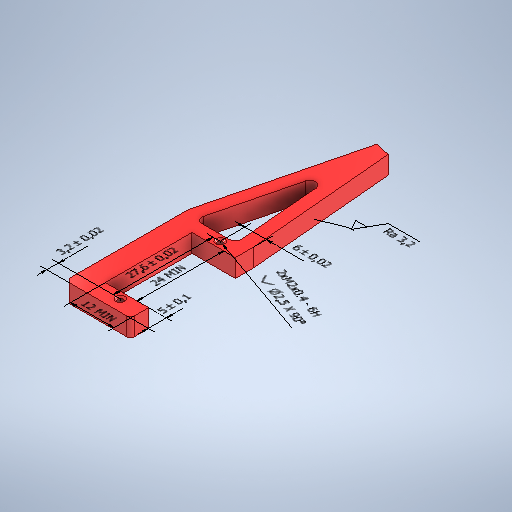
# Autodesk Inventor part: CAM3D
Saved by Autodesk Inventor 2025 (Build 290162000, 162)
## iProperties
Created: 2023-06-22
Part Number: CAM3D
Material: EN AW-6060 T6
Document SubType Name: Modeling
Designer: Roman
Density: 2.7 g/cm^3
Appearance: Light Red
Mass: 15.4015 g
Surface Area: 41.4189 cm^2
Volume: 5.70428 cm^3
Description: Přední noha
Polotovar: KR...
Author: Roman
## iProperties of the stored document CAM3D_3D tisk.ipt
Created: 2024-11-28
Part Number: CAM3D_3D tisk
Material: Všeobecné
Document SubType Name: Modeling
Designer: s21suk
Density: 1 g/cm^3
Appearance: Výchozí
Author: s21suk
## iProperties of the stored document MemberDocs/xIbcejt23Mcnw1njhJ3dlasc4Ob
Created: 2023-06-22
Part Number: CAM3D
Material: EN AW-6060 T6
Document SubType Name: Modeling
Designer: Roman
Density: 2.7 g/cm^3
Appearance: Light Red
Mass: 15.4015 g
Surface Area: 41.4189 cm^2
Volume: 5.70428 cm^3
Description: Přední noha
Polotovar: KR...
Author: Roman
Autodesk Inventor part; units mm, degrees
ref_plane "YZ Plane" through (0, 0, 0) normal (1, 0, 0) x (0, 1, 0)
ref_plane "XZ Plane" through (0, 0, 0) normal (0, 1, 0) x (-1, 0, 0)
ref_plane "XY Plane" through (0, 0, 0) normal (0, 0, 1) x (1, 0, 0)
sketch "Sketch1" plane through (0, 0, 0) normal (0, 1, 0) x (-1, 0, 0)
  line L0 (0, 0) -> (18, 0)
  line L1 (0, 0) -> (0, -5)
  line L2 (0, -5) -> (3.5719, -45.8274)
  line L3 (18, 0) -> (18, -5)
  line L4 (18, -5) -> (7.5719, -46.8247)
  line L5 (3.5719, -45.8274) -> (7.5719, -46.8247)
  dimension "d0" = 18
  dimension "d1" = 5
  dimension "d3" = 175
  dimension "d6" = 76
  dimension "d7" = 4
  constraints: 12 end point, 2 vertical, 1 horizontal, 1 parallel, 1 perpendicular
  measures "d0" distance of L0.start L0.end
  measures "d1" distance of L0.start L1.end
  measures "d3" angle of L2 L1
  measures "d6" angle of L0 L4
  measures "d7" horizontal distance of L2.end L4.end
extrude "Extrusion1" add sketch "Sketch1" along normal blind 5
shell "Shell1" thickness 3.5 removed faces 2 at (-7.1906, 5, -18.6091) at (-7.1906, 0, -18.6091)
fillet "Fillet1" radius 1.5875 5 edges at (-3.5, 2.5, -4.8472) (-6.3393, 2.5, -37.3009) (-3.5, 2.5, -3.5) (-14.5, 2.5, -3.5) (-14.5, 2.5, -4.5703)
sketch "Sketch2" plane through (0, 0, 0) normal (0, -1, 0) x (1, 0, 0)
  line L0 (0, 0) -> (-12, 0)
  line L1 (-12, 0) -> (-12, 24)
  line L2 (-12, 24) -> (0, 24)
  line L3 (0, 24) -> (0, 0)
  line L4 (0, 24) -> (-12, 24)
  line L5 (-12, 24) -> (-12, 29)
  line L6 (-12, 29) -> (0, 29)
  line L7 (0, 29) -> (0, 24)
  line L8 (-12, 0) -> (-18, 0)
  line L9 (-18, 0) -> (-18, 24)
  line L10 (-18, 24) -> (-12, 24)
  line L11 (-12, 24) -> (-12, 0)
  line L12 (-18, 24) -> (-13.7574, 24) construction
  line L13 (-12, 29) -> (-16.8, 29)
  line L14 (-16.8, 29) -> (-18, 27.8)
  line L15 (-18, 27.8) -> (-18, 24)
  dimension "d14" = 24
  dimension "d15" = 5
  dimension "d16" = 12
  dimension "d18" = 6
  dimension "d57" = 1.2
  dimension "d58" = 135
  constraints: 32 end point, 6 parallel, 5 horizontal, 4 perpendicular, 2 collinear
  measures "d14" distance of L0.end L1.end
  measures "d15" distance of L4.end L5.end
  measures "d16" distance between parallel lines of L7 L5
  measures "d18" distance between parallel lines of L9 L1
  measures "d57" horizontal distance of L14.end L13.end
  measures "d58" angle of L13 L14
extrude "Extrusion2" add sketch "Sketch2" against normal blind 5 contours L8 L9 L10 L1 | L2 L5 L6 L7 | L10 L15 L14 L13 L5
fillet "Fillet3" radius 1 1 edges at (0, 2.5, 29)
sketch "Sketch4" plane through (0, 5, 0) normal (0, 1, 0) x (1, 0, 0)
  line L0 (-12, -24) -> (-12, 0) projected
  line L1 (-12, -12) -> (-18, -12)
  line L2 (-18, 5) -> (-18, -29) projected
  line L3 (0, -24) -> (-12, -24) projected
  line L4 (-12, 0) -> (0, 0) projected
  circle A0 centre (-6, -25.8) radius 0.8
  circle A1 centre (-6, 1.8) radius 0.8
  line L5 (0, -28) -> (0, -24) projected
  point P0 (-18, 1.9304)
  point P1 (-18, -27.8)
  point P2 (-16.8, -29)
  dimension "d31" = 1.6
  dimension "d32" = 27.6
  dimension "d43" = 6
  dimension "d46" = 13.8
  constraints: 2 centre point, 2 end point, 1 horizontal, 1 midpoint, 1 symmetric about line, 3 other
  measures "d31" diameter of A0
  measures "d32" distance of A1.centre A0.centre
  measures "d43" horizontal distance of L0.start A0.centre
  measures "d46" vertical distance of A0.centre L1.end
hole "Hole1" at (-6, 5, 25.8) at (-6, 5, -1.8) direction (0, -1, 0) diameter 1.567 depth 10 countersink diameter 2.5 countersink angle 90 thread size "M2x0.4" class "6H" standard "ISO Metric profile"
sketch "Sketch17" plane through (0, 5, 0) normal (0, 1, 0) x (1, 0, 0)
  line L0 (-15.0964, 25.5) -> (0.714, 25.5)
  line L1 (-12, 0) -> (0, 0) projected
  line L2 (-5.1146, 3.5) -> (-12.7349, 3.5) projected
  line L3 (0.714, 25.5) -> (-0.9097, 44.0597)
  line L4 (-15.0964, 25.5) -> (-10.3033, 44.7241)
  line L5 (0, 5) -> (-3.5719, 45.8274) projected
  line L6 (-7.5719, 46.8247) -> (-18, 5) projected
  line L7 (-4.6811, 48.4754) -> (-4.2422, 48.3659)
  line L8 (-3.5719, 45.8274) -> (-7.5719, 46.8247) projected
  arc A0 (-0.9097, 44.0597) -> (-4.6811, 48.4754) centre (-5.8907, 43.6239) ccw
  arc A1 (-4.2422, 48.3659) -> (-10.3033, 44.7241) centre (-5.4518, 43.5145) ccw
  point P0 (-8.9248, 3.5)
  point P1 (-4.4629, 48.4157)
  dimension "d152" = 22
  dimension "d153" = 2.498
  dimension "d154" = 2.142
  dimension "d155" = 2.301
  dimension "d156" = 5
  constraints: 8 end point, 4 point on circle, 4 tangent, 3 parallel, 2 centre point, 1 equal radius, 1 horizontal, 1 midpoint
  measures "d152" distance from line of L0 point (-8.925, 3.5)
  measures "d153" distance between parallel lines of L5 L3
  measures "d154" distance between parallel lines of L4 L6
  measures "d155" distance between parallel lines of L8 L7
  measures "d156" radius of A0
extrude "Extrusion13" [suppressed]
sketch "Sketch18" plane through (-15.4653, 7.5, -25.5) normal (0, 0, 1) x (1, 0, 0)
  line L0 (16.1813, -10) -> (16.1813, 0) construction
  line L1 (4.8628, 0) -> (0, 0) construction
  line L2 (16.1813, -10) -> (0, 0) construction
  line L3 (0, -10) -> (0, 0) construction
  line L4 (16.1813, 0) -> (0, -10) construction
  line L5 (23.0907, 2.5) -> (-6.9093, 2.5)
  line L6 (-6.9093, 2.5) -> (-6.9093, -12.5)
  line L7 (-6.9093, -12.5) -> (23.0907, -12.5)
  line L8 (23.0907, -12.5) -> (23.0907, 2.5)
  line L9 (23.0907, 2.5) -> (-6.9093, -12.5) construction
  line L10 (-6.9093, 2.5) -> (23.0907, -12.5) construction
  point P0 (15.4653, -7.5)
  point P1 (8.0907, -5)
  dimension "d161" = 25
  dimension "d162" = 15
  constraints: 16 end point, 3 midpoint, 2 parallel, 1 horizontal, 1 perpendicular
  measures "d162" distance of L6.end L5.end
extrude "Extrusion14" [suppressed]
combine "Combine8" [suppressed]
extrude "Extrusion15" [suppressed]
combine "Combine9" [suppressed]
combine "Combine10" [suppressed]
sketch "Sketch20" plane through (-15.4653, 7.5, -21.5) normal (0, 0, 1) x (1, 0, 0)
  line L0 (10.1584, -7.5) -> (13.6718, -7.5) projected
  line L1 (6.1837, -2.5) -> (2.5765, -2.5) projected
  line L2 (11.871, -7.5) -> (3.871, -7.5)
  line L3 (3.871, -7.5) -> (3.871, -2.5)
  line L4 (3.871, -2.5) -> (11.871, -2.5)
  line L5 (11.871, -2.5) -> (11.871, -7.5)
  circle A0 centre (19.0907, -8.5) radius 1
  line L6 (23.0907, -12.5) -> (-6.9093, -12.5) construction
  circle A1 centre (-2.9093, -1.5) radius 1
  line L7 (23.0907, -12.5) -> (23.0907, 2.5) construction
  line L8 (23.0907, 2.5) -> (-6.9093, 2.5) construction
  line L9 (11.871, -7.5) -> (3.871, -7.5)
  line L10 (3.871, -7.5) -> (3.871, -10)
  line L11 (3.871, -10) -> (11.871, -10)
  line L12 (11.871, -10) -> (11.871, -7.5)
  line L13 (11.871, -2.5) -> (3.871, -2.5)
  line L14 (3.871, -2.5) -> (3.871, 0)
  line L15 (3.871, 0) -> (11.871, 0)
  line L16 (11.871, 0) -> (11.871, -2.5)
  line L17 (-6.9093, 2.5) -> (-6.9093, -12.5) projected
  point P0 (15.4653, -7.5)
  point P1 (23.0907, -5)
  point P2 (23.0907, -5)
  dimension "d167" = 9.224
  dimension "d168" = 3.5943
  dimension "d171" = 2
  dimension "d173" = 7.5
  dimension "d175" = 4.22
  dimension "d181" = 2.5
  dimension "d185" = 8
  dimension "d186" = 2.5
  dimension "d202" = 15
  dimension "d203" = 11
  dimension "d204" = 3.561
  dimension "d205" = 2
  constraints: 24 end point, 6 parallel, 3 horizontal, 3 perpendicular, 2 centre point, 2 midpoint, 2 point on line, 1 collinear
  measures "d168" distance from line of L5 point (15.465, -7.5)
  measures "d171" diameter of A0
  measures "d181" distance of L10.end L9.end
  measures "d185" distance of L14.end L15.end
  measures "d186" distance of L13.end L14.end
  measures "d202" distance between parallel lines of L6 L8
  measures "d205" diameter of A1
extrude "Extrusion16" [suppressed]
extrude "Extrusion17" [suppressed]
chamfer "Chamfer2" [suppressed]
chamfer "Chamfer3" [suppressed]
chamfer "Chamfer4" [suppressed]
chamfer "Chamfer5" [suppressed]
sketch "Sketch21" plane through (-15.4653, 7.5, -25.5) normal (0, 0, 1) x (1, 0, 0)
  line L0 (23.0907, 2.5) -> (-6.9093, 2.5) projected
  line L1 (-6.9093, 2.5) -> (-6.9093, -10.5) projected
  line L2 (23.0907, 2.5) -> (-6.9093, 2.5)
  line L3 (-6.9093, 2.5) -> (-6.9093, -5)
  line L4 (-6.9093, -5) -> (23.0907, -5)
  line L5 (23.0907, -5) -> (23.0907, 2.5)
  point P0 (15.4653, -7.5)
  dimension "d194" = 7.5
  constraints: 8 end point, 2 parallel, 1 horizontal, 1 perpendicular, 1 point on line
  measures "d194" distance of L3.end L2.end
extrude "Extrusion18" [suppressed]
extrude "Extrusion19" [suppressed]
combine "Combine11" [suppressed]
sketch "Sketch22" plane through (-15.4653, 7.5, -25.5) normal (0, 0, 1) x (1, 0, 0)
  circle A0 centre (-2.9093, -1.5) radius 1 construction
  line L0 (-2.9093, -2.5) -> (-2.9093, -1.5) construction
  circle A1 centre (-2.9093, -1.5) radius 1
  point P0 (15.4653, -7.5)
  constraints: 2 end point, 2 vertical alignment, 1 coincident, 1 vertical, 3 other
extrude "Extrusion20" [suppressed]
chamfer "Chamfer7" [suppressed]
sketch "Sketch23" plane through (7.6254, 10, -60.5) normal (0, 0, -1) x (-1, 0, 0)
  line L0 (30, -7.5) -> (3.5, -7.5) projected
  line L1 (30, -7.5) -> (30, -11)
  line L2 (26.5, -7.5) -> (30, -11) projected
  line L3 (30, -11) -> (26.5, -7.5)
  line L4 (26.5, -7.5) -> (30, -7.5)
  line L5 (0, -4) -> (3.5, -7.5) projected
  line L6 (3.5, -7.5) -> (0, -7.5)
  line L7 (0, -7.5) -> (0, -4)
  line L8 (0, -4) -> (3.5, -7.5)
  point P0 (7.6254, -10)
  constraints: 12 end point, 2 collinear, 2 perpendicular, 1 point on line
extrude "Extrusion21" [suppressed]
extrude "Extrusion22" [suppressed]
combine "Combine12" [suppressed]
combine "Combine13" [suppressed]
fillet "Fillet6" [suppressed]
sketch "Sketch24" plane through (-22.3746, 10, -25.5) normal (0, 1, 0) x (1, 0, 0)
  circle A0 centre (24, 29) radius 1
  line L0 (30, 35) -> (0, 35) projected
  line L1 (30, 0) -> (30, 35) projected
  circle A1 centre (24, 11) radius 1
  circle A2 centre (6, 29) radius 1
  circle A3 centre (6, 11) radius 1
  point P0 (22.3746, -25.5)
  dimension "d216" = 2
  dimension "d217" = 4.064
  dimension "d218" = 4.147
  dimension "d221" = 18
  dimension "d224" = 20
  constraints: 4 centre point, 1 horizontal, 1 vertical, 6 other
  measures "d216" diameter of A0
  measures "d221" distance of A0.centre A1.centre
extrude "Extrusion23" [suppressed]
extrude "Extrusion24" [suppressed]
chamfer "Chamfer8" [suppressed]
chamfer "Chamfer9" [suppressed]
body "Solid1"
body "Solid9"
body "Solid10"
body "Solid11"
body "Solid12"
body "Solid13"
body "Solid14"
